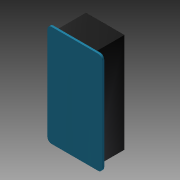
# Autodesk Inventor part: Digit Display
Saved by Autodesk Inventor 2015 (Build 190159000, 159)
## iProperties
Created: 2016-02-20
Part Number: Digit Display
Material: Generic
Document SubType Name: Modeling
Designer: 23902
Density: 1 g/cm^3
Appearance: Default
Author: 23902
Autodesk Inventor part; units mm, degrees
ref_plane "YZ Plane" through (0, 0, 0) normal (1, 0, 0) x (0, 1, 0)
ref_plane "XZ Plane" through (0, 0, 0) normal (0, 1, 0) x (-1, 0, 0)
ref_plane "XY Plane" through (0, 0, 0) normal (0, 0, 1) x (1, 0, 0)
sketch "Sketch1" plane through (0, 0, 0) normal (0, 1, 0) x (-1, 0, 0)
  line L0 (-13.5, 25) -> (-13.5, -25)
  line L1 (-13.5, -25) -> (13.5, -25)
  line L2 (13.5, -25) -> (13.5, 25)
  line L3 (13.5, 25) -> (-13.5, 25)
  line L4 (-13.5, 25) -> (13.5, -25) construction
  line L5 (-13.5, -25) -> (13.5, 25) construction
  point P0 (0, 0)
  dimension "d0" = 50
  dimension "d1" = 27
  constraints: 12 end point, 2 midpoint, 2 parallel, 1 perpendicular, 1 vertical
  measures "d0" distance of L0.start L0.end
  measures "d1" distance of L1.end L0.end
extrude "Extrusion1" add sketch "Sketch1" along normal blind 1
fillet "Fillet1" radius 2 4 edges at (13.5, 0.5, 25) (-13.5, 0.5, 25) (-13.5, 0.5, -25) (13.5, 0.5, -25)
sketch "Sketch2" plane through (0, 1, 0) normal (0, 1, 0) x (1, 0, 0)
  line L0 (9.5, -24.5) -> (9.5, 24.5)
  line L1 (9.5, 24.5) -> (-9.5, 24.5)
  line L2 (-9.5, 24.5) -> (-9.5, -24.5)
  line L3 (-9.5, -24.5) -> (9.5, -24.5)
  line L4 (9.5, -24.5) -> (-9.5, 24.5) construction
  line L5 (9.5, 24.5) -> (-9.5, -24.5) construction
  point P0 (0, 0)
  dimension "d5" = 49
  dimension "d6" = 19
  constraints: 12 end point, 2 midpoint, 2 parallel, 1 perpendicular, 1 vertical
  measures "d5" distance of L0.start L0.end
  measures "d6" distance of L1.end L0.end
extrude "Extrusion2" add sketch "Sketch2" along normal blind 14
sketch "Sketch3" plane through (0, 15, 0) normal (0, 1, 0) x (1, 0, 0)
  point P0 (0, 0)
sketch "Sketch4" plane through (0, 15, 0) normal (0, 1, 0) x (1, 0, 0)
  line L0 (-9.2797, -24.5843) -> (-9.5, 24.5) construction
  line L1 (-9.5, 24.5) -> (9.2797, 24.5843) construction
  line L2 (9.2797, 24.5843) -> (9.5, -24.5) construction
  line L3 (9.5, -24.5) -> (-9.2797, -24.5843) construction
  line L4 (9.5, -24.5) -> (9.5, 24.5) projected
  line L5 (9.5, 24.5) -> (-9.5, 24.5) projected
  line L6 (-9.5, 24.5) -> (-9.5, -24.5) projected
  line L7 (-9.5, -24.5) -> (9.5, -24.5) projected
  point P0 (0, 0)
  constraints: 2 coincident, 2 other
decal "Decal1"
body "Solid1"
